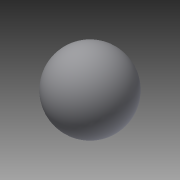
# Autodesk Inventor part: Ball
Saved by Autodesk Inventor 2014 (Build 180170000, 170)
## iProperties
Created: 2016-01-25
Part Number: Ball
Material: Generic
Document SubType Name: Modeling
Designer: CAD
Density: 1 g/cm^3
Appearance: Default
Author: CAD
Autodesk Inventor part; units mm, degrees
ref_plane "XY Plane" through (0, 0, 0) normal (0, 0, 1) x (1, 0, 0)
sketch "Sketch1" plane through (0, 0, 0) normal (0, 1, 0) x (-1, 0, 0)
  circle A0 centre (0, 0) radius 127
  line L0 (31.6782, -122.9858) -> (-31.6782, 122.9858)
  dimension "d0" = 254
  constraints: 2 end point, 2 point on circle, 1 centre point, 1 coincident, 1 midpoint
  measures "d0" diameter of A0
revolve "Revolution1" add sketch "Sketch1" angle 360 about axis through (-31.6782, 0, -122.9858) along (0.2494343, 0, 0.9683917) picked at (76.7989, -23.9961) contours A0 L0
ref_plane "Work Plane2" through (0, -127, 0) normal (0, 1, 0) x (-1, 0, 0)
ref_plane "Work Plane1" through (0, 127, 0) normal (0, 1, 0) x (-1, 0, 0)
ref_plane "Work Plane3" through (127, 0, 0) normal (1, 0, 0) x (0, 1, 0)
ref_plane "Work Plane5" through (-127, 0, 0) normal (1, 0, 0) x (0, 1, 0)
body "Solid1"
